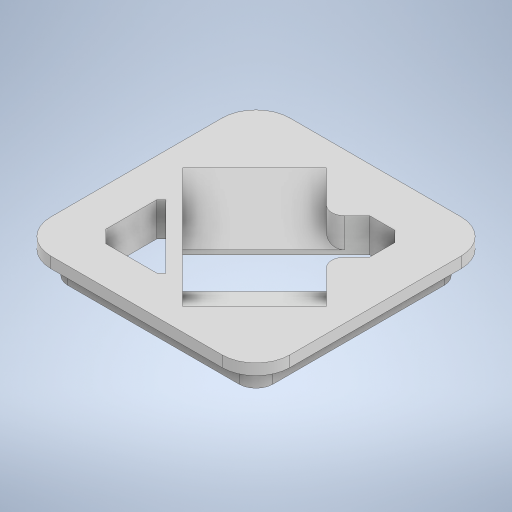
# Autodesk Inventor part: pieza_edu_fisica
Saved by Autodesk Inventor 2024 (Build 280153000, 153)
## iProperties
Created: 2023-06-29
Part Number: pieza_edu_fisica
Material: Generic
Document SubType Name: Modeling
Designer: LabTel_Admin
Density: 1 g/cm^3
Appearance: Default
Author: LabTel_Admin
Autodesk Inventor part; units mm, degrees
ref_plane "YZ Plane" through (0, 0, 0) normal (1, 0, 0) x (0, 1, 0)
ref_plane "XZ Plane" through (0, 0, 0) normal (0, 1, 0) x (-1, 0, 0)
ref_plane "XY Plane" through (0, 0, 0) normal (0, 0, 1) x (1, 0, 0)
sketch "Sketch1" plane through (0, 0, 0) normal (0, 1, 0) x (-1, 0, 0)
  line L0 (-10.105, -14.105) -> (10.105, -14.105)
  line L1 (14.105, -10.105) -> (14.105, 10.105)
  line L2 (10.105, 14.105) -> (-10.105, 14.105)
  line L3 (-14.105, 10.105) -> (-14.105, -10.105)
  line L4 (-14.105, -14.105) -> (14.105, 14.105) construction
  line L5 (14.105, -14.105) -> (-14.105, 14.105) construction
  arc A0 (14.105, 10.105) -> (10.105, 14.105) centre (10.105, 10.105) ccw
  arc A1 (-10.105, 14.105) -> (-14.105, 10.105) centre (-10.105, 10.105) ccw
  arc A2 (-14.105, -10.105) -> (-10.105, -14.105) centre (-10.105, -10.105) ccw
  arc A3 (10.105, -14.105) -> (14.105, -10.105) centre (10.105, -10.105) ccw
  line L6 (10.105, 14.105) -> (10.105, 8.105) construction
  line L7 (9.605, 8.105) -> (9.605, 2.105)
  line L8 (8.105, 9.605) -> (2.105, 9.605)
  line L9 (8.105, 9.605) -> (9.605, 8.105)
  line L10 (8.9013, 1.7376) -> (1.5695, 9.0695)
  line L11 (2.105, 9.605) -> (1.5695, 9.0695)
  line L12 (8.9013, 1.7376) -> (9.0695, 1.5695)
  line L13 (9.605, 2.105) -> (9.0695, 1.5695)
  line L14 (8.0814, 0.5776) -> (0.5776, 8.0814)
  line L15 (2.2082, 6.4508) -> (-8.8227, -4.58)
  line L16 (6.4508, 2.2082) -> (-4.58, -8.8227)
  line L17 (-4.58, -8.8227) -> (-7.58, -8.8227)
  line L18 (-8.8227, -4.58) -> (-8.8227, -7.58)
  line L19 (-8.8227, -7.58) -> (-7.58, -8.8227)
  line L20 (-10.105, 12.105) -> (10.105, 12.105)
  arc A4 (12.105, 10.105) -> (10.105, 12.105) centre (10.105, 10.105) ccw
  line L21 (12.105, 10.105) -> (12.105, -10.105)
  arc A5 (10.105, -12.105) -> (12.105, -10.105) centre (10.105, -10.105) ccw
  line L22 (10.105, -12.105) -> (-10.105, -12.105)
  arc A6 (-12.105, -10.105) -> (-10.105, -12.105) centre (-10.105, -10.105) ccw
  line L23 (-12.105, -10.105) -> (-12.105, 10.105)
  arc A7 (-10.105, 12.105) -> (-12.105, 10.105) centre (-10.105, 10.105) ccw
  point P0 (0, 0)
  point P1 (8.855, 8.855)
  point P2 (4.3295, 4.3295)
  dimension "d0" = 28.21
  dimension "d1" = 28.21
  dimension "d2" = 4
  dimension "d13" = 6
  dimension "d16" = 6
  dimension "d18" = 5
  dimension "d21" = 1.4
  dimension "d22" = 15.6
  dimension "d24" = 3
  dimension "d25" = 3
  dimension "d28" = 2
  constraints: 48 end point, 16 point on circle, 9 point on line, 8 centre point, 8 tangent, 6 parallel, 6 perpendicular, 4 midpoint, 3 equal radius, 3 horizontal, 3 symmetric about line, 2 vertical, 7 other
  measures "d0" distance of L5.end L4.end
  measures "d1" distance of L4.end L5.start
  measures "d2" radius of A0
  measures "d13" distance of L7.start L7.end
  measures "d16" distance of L8.start L8.end
  measures "d18" distance from line of L10 point (8.855, 8.855)
  measures "d21" distance between parallel lines of L14 L10
  measures "d22" distance of L15.start L15.end
  measures "d24" distance of point (4.33, 4.33) L15.start
  measures "d25" distance of L16.end L17.end
  measures "d28" distance between parallel lines of L2 L20
extrude "Extrusion5" add sketch "Sketch1" against normal blind 1.3 contours A2 L3 A1 L2 A0 L1 A3 L0
extrude "Extrusion6" add sketch "Sketch1" against normal blind 4 contours L20 A4 L21 A5 L22 A6 L23 A7
sketch "Sketch5" plane through (-2.2082, -4, 6.4508) normal (0.7071068, 0, -0.7071068) x (-0.7071068, 0, -0.7071068)
  line L0 (6, 0) -> (0, 0) projected
  line L1 (6, 0) -> (0, 0)
  line L2 (0, 0) -> (0, 0.5)
  line L3 (0, 0.5) -> (6, 0.5)
  line L4 (6, 0.5) -> (6, 0)
  point P0 (3, 4)
  dimension "d33" = 6
  dimension "d34" = 0.5
  constraints: 8 end point, 2 parallel, 1 horizontal, 1 perpendicular
  measures "d33" distance of L2.end L3.end
  measures "d34" distance of L1.end L2.end
extrude "Extrusion7" cut sketch "Sketch5" against normal blind 4
sketch "Sketch6" plane through (0, 0, 0) normal (0, 1, 0) x (1, 0, 0)
  line L0 (-14.105, -14.105) -> (14.105, 14.105) construction
  line L1 (-14.105, 14.105) -> (14.105, -14.105) construction
  line L2 (-9.0695, -1.5695) -> (-1.5695, -9.0695) projected
  line L3 (2.8146, -11.4736) -> (11.2999, -2.9883)
  line L4 (1.1859, 7.1256) -> (-2.8423, 11.1538)
  line L5 (-2.8423, 11.1538) -> (-11.3275, 2.6685)
  line L6 (4.58, 8.8227) -> (7.58, 8.8227) projected
  line L7 (-6.4508, -2.2082) -> (4.58, 8.8227) projected
  line L8 (11.2999, -2.9883) -> (7.1256, 1.1859)
  line L9 (-2.2082, -6.4508) -> (-6.4508, -2.2082) projected
  line L10 (-2.2082, -6.4508) -> (2.8146, -11.4736)
  line L11 (-6.4508, -2.2082) -> (-11.3275, 2.6685)
  line L12 (8.8227, 4.58) -> (-2.2082, -6.4508) projected
  line L13 (7.1256, 1.1859) -> (6.9842, 1.3273)
  line L14 (1.1859, 7.1256) -> (1.3273, 6.9842)
  line L15 (6.2771, 2.0344) -> (-2.2082, -6.4508)
  line L16 (2.0344, 6.2771) -> (-6.4508, -2.2082)
  line L17 (6.9842, 1.3273) -> (6.2771, 2.0344)
  line L18 (1.3273, 6.9842) -> (2.0344, 6.2771)
  point P0 (0, 0)
  dimension "d39" = 20
  dimension "d53" = 12
  constraints: 28 end point, 9 perpendicular, 7 point on line, 1 collinear, 1 parallel, 1 symmetric about line
  measures "d39" distance of L4.end L3.end
  measures "d53" distance of L4.end L5.end
extrude "Extrusion8" cut sketch "Sketch6" against normal through all
sketch "Sketch8" plane through (11.2999, -4, 2.9883) normal (-0.7071068, 0, 0.7071068) x (0.7071068, 0, 0.7071068)
  line L0 (0, 0) -> (-7.1033, 0) projected
  line L1 (0, 4) -> (0, 0) projected
  line L2 (0, 4) -> (0, 0)
  line L3 (0, 0) -> (-7.1033, 0)
  line L4 (-20, 4) -> (-20, 0) projected
  line L5 (-20, 4) -> (-20, 0)
  line L6 (-13.1033, 0) -> (-20, 0) projected
  line L7 (-13.0928, 0) -> (-20, 0)
  line L8 (-13.1033, 0) -> (-13.1033, 0.5)
  line L9 (-13.1033, 4) -> (-13.1033, 0) projected
  line L10 (-13.1033, 0.5) -> (-20, 4)
  line L11 (-7.1033, 0) -> (-7.1033, 0.5)
  line L12 (-7.1033, 0.5) -> (0, 4)
  point P0 (-10.1033, 4)
  point P1 (-13.1033, 0)
  dimension "d48" = 0.5
  dimension "d49" = 0.5
  constraints: 16 end point, 3 collinear, 2 perpendicular, 2 point on line
  measures "d48" distance of L6.start L8.end
  measures "d49" distance of L0.end L11.end
extrude "Extrusion10" add sketch "Sketch8" along normal blind 12
fillet "Fillet2" radius 1.5 2 edges at (2.0344, -1.75, -6.2771) (6.2771, -1.75, -2.0344)
body "Solid3"
